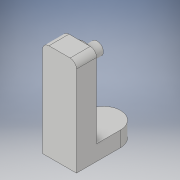
# Autodesk Inventor part: Waist Link-lrg
Saved by Autodesk Inventor 2017 (Build 210142000, 142)
## iProperties
Created: 2017-05-25
Part Number: Waist Link-lrg
Material: Generic
Document SubType Name: Modeling
Designer: garre
Density: 1 g/cm^3
Appearance: Default
Author: garre
Autodesk Inventor part; units mm, degrees
ref_plane "YZ Plane" through (0, 0, 0) normal (1, 0, 0) x (0, 1, 0)
ref_plane "XZ Plane" through (0, 0, 0) normal (0, 1, 0) x (-1, 0, 0)
ref_plane "XY Plane" through (0, 0, 0) normal (0, 0, 1) x (1, 0, 0)
sketch "Sketch1" plane through (0, 0, 0) normal (0, 1, 0) x (-1, 0, 0)
  line L0 (0, 0) -> (162.56, 0)
  line L1 (162.56, 0) -> (162.56, -210.82)
  line L2 (81.28, -292.1) -> (81.28, -292.1)
  line L3 (0, -210.82) -> (0, 0)
  arc A0 (81.28, -292.1) -> (162.56, -210.82) centre (81.28, -210.82) ccw
  arc A1 (0, -210.82) -> (81.28, -292.1) centre (81.28, -210.82) ccw
  point P0 (162.56, -292.1)
  point P1 (0, -292.1)
  dimension "d0" = 292.1
  dimension "d1" = 162.56
  dimension "d2" = 81.28
  constraints: 8 end point, 4 point on circle, 4 point on line, 4 tangent, 2 centre point, 2 parallel, 1 concentric, 1 horizontal, 1 perpendicular
  measures "d0" distance of L0.end point (162.56, -292.1)
  measures "d1" distance of point (162.56, -292.1) point (0, -292.1)
  measures "d2" radius of A0
extrude "Extrusion1" add sketch "Sketch1" along normal blind 73.66
sketch "Sketch2" plane through (0, 73.66, 0) normal (0, 1, 0) x (1, 0, 0)
  line L0 (-162.56, 0) -> (0, 0) projected
  line L1 (0, 0) -> (0, 210.82) projected
  line L2 (-162.56, 0) -> (0, 0)
  line L3 (0, 0) -> (0, 96.52)
  line L4 (0, 96.52) -> (-162.56, 96.52)
  line L5 (-162.56, 96.52) -> (-162.56, 0)
  dimension "d23" = 114.3
  constraints: 8 end point, 2 parallel, 1 horizontal, 1 perpendicular, 1 point on line
  measures "d23" distance from line of L1.end L4
extrude "Extrusion2" add sketch "Sketch2" along normal blind 388.62
sketch "Sketch3" plane through (-162.56, 0, 0) normal (0, 0, 1) x (1, 0, 0)
  line L0 (162.56, 0) -> (0, 0) projected
  line L1 (162.56, 0) -> (162.56, 462.28) projected
  line L2 (0, 0) -> (162.56, 0)
  line L3 (162.56, 0) -> (162.56, 431.8)
  line L4 (132.08, 462.28) -> (30.48, 462.28)
  line L5 (0, 431.8) -> (0, 0)
  arc A0 (30.48, 462.28) -> (0, 431.8) centre (30.48, 431.8) ccw
  arc A1 (162.56, 431.8) -> (132.08, 462.28) centre (132.08, 431.8) ccw
  dimension "d8" = 30.48
  constraints: 8 end point, 4 point on circle, 4 tangent, 2 centre point, 2 parallel, 2 point on line, 1 equal radius, 1 horizontal, 1 perpendicular
  measures "d8" radius of A0
extrude "Extrusion3" cut sketch "Sketch3" against normal blind 508 keep common part
sketch "Sketch4" plane through (0, 73.66, -96.52) normal (0, 0, -1) x (-1, 0, 0)
  line L0 (132.08, 388.62) -> (30.48, 388.62) projected
  circle A0 centre (81.28, 313.69) radius 59.69
  line L1 (0, -73.66) -> (162.56, -73.66) projected
  dimension "d12" = 119.38
  dimension "d22" = 387.35
  constraints: 1 centre point
  measures "d12" diameter of A0
  measures "d22" distance from line of L1 A0.centre
extrude "Extrusion4" add sketch "Sketch4" along normal blind 20.32
sketch "Sketch5" plane through (-81.28, 387.35, -116.84) normal (0, 0, -1) x (-1, 0, 0)
  circle A0 centre (0, 0) radius 29.845
  point P0 (-81.28, -387.35)
  dimension "d15" = 59.69
  constraints: 1 centre point
  measures "d15" diameter of A0
extrude "Extrusion5" add sketch "Sketch5" along normal blind 63.5
sketch "Sketch6" plane through (0, 0, 0) normal (0, -1, 0) x (1, 0, 0)
  arc A0 (-162.56, -210.82) -> (0, -210.82) centre (-81.28, -210.82) ccw projected
  circle A1 centre (-81.28, -210.82) radius 38.1
  point P0 (0, 0)
  dimension "d18" = 76.2
  constraints: 1 centre point, 1 coincident
  measures "d18" diameter of A1
extrude "Extrusion6" cut sketch "Sketch6" against normal blind 25.4
body "Solid1"
